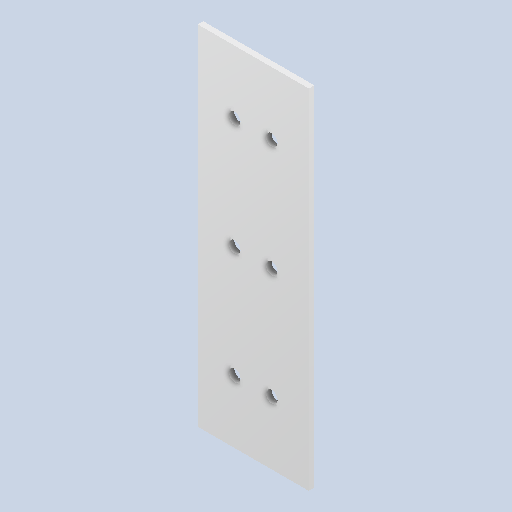
# Autodesk Inventor part: rail_rail
Saved by Autodesk Inventor 2024.1 (Build 281209000, 209)
## iProperties
Created: 2025-01-17
Part Number: rail_rail
Material: アルミニウム 6061
Document SubType Name: Sheet Metal
Designer: hibik
Density: 2.7 g/cm^3
Sheet Metal Rule: Default_mm
Appearance: アルミニウム - フラット
Author: hibik
Autodesk Inventor part; units mm, degrees
ref_plane "YZ Plane" through (0, 0, 0) normal (1, 0, 0) x (0, 1, 0)
ref_plane "XZ Plane" through (0, 0, 0) normal (0, 1, 0) x (-1, 0, 0)
ref_plane "XY Plane" through (0, 0, 0) normal (0, 0, 1) x (1, 0, 0)
sketch "スケッチ1" plane through (0, 0, 0) normal (0, 0, 1) x (1, 0, 0)
  line L0 (0, 0) -> (30, 0)
  line L1 (30, 0) -> (30, 94)
  line L2 (30, 94) -> (0, 94)
  line L3 (0, 94) -> (0, 0)
  dimension "d0" = 30
  dimension "d1" = 94
  measures "d0" distance of L2.end L1.end
  measures "d1" distance of L1.end L0.end
extrude "プレート1" add sketch "スケッチ1" along normal blind 1.5
sketch "スケッチ2" plane through (0, 0, 1.5) normal (0, 0, 1) x (1, 0, 0)
  line L0 (30, 94) -> (30, 0) projected
  circle A0 centre (10, 47) radius 1.6
  circle A1 centre (20, 47) radius 1.6
  line L1 (30, 0) -> (0, 0) projected
  line L2 (30, 94) -> (30, 0) projected
  line L3 (0, 94) -> (30, 94) projected
  line L4 (0, 0) -> (0, 94) projected
  line L5 (15, 94) -> (15, 0)
  circle A2 centre (20, 17) radius 1.6
  circle A3 centre (10, 17) radius 1.6
  circle A4 centre (20, 77) radius 1.6
  circle A5 centre (10, 77) radius 1.6
  circle A6 centre (20, 47) radius 1.6
  circle A7 centre (10, 47) radius 1.6
  point P0 (30, 47)
  dimension "d3" = 3.2
  dimension "d4" = 3.2
  dimension "d5" = 10
  dimension "d8" = 30
  dimension "d11" = 30
  constraints: 8 centre point, 3 midpoint, 2 end point, 2 vertical, 1 horizontal alignment, 1 symmetric about line, 12 other
  measures "d3" diameter of A0
  measures "d4" diameter of A1
  measures "d5" distance of A1.centre A0.centre
  measures "d8" distance of A1.centre A2.centre
  measures "d11" distance of A1.centre A4.centre
extrude "切り取り1" cut sketch "スケッチ2" against normal blind 1.5 contours A0 | A1 | A2 | A3 | A4 | A5
equation "\"d14\" = Thickness"
equation "\"d2\" = Thickness"
equation "\"BendRadius\" = Thickness"
equation "\"BendReliefWidth\" = Thickness"
equation "\"BendReliefDepth\" = 0.5 * Thickness"
equation "\"CornerReliefSize\" = 4 * Thickness"
equation "\"MinimumRemnant\" = 2 * Thickness"
equation "\"TransitionRadius\" = BendRadius"
equation "\"JacobiRadiusSize\" = BendRadius"
equation "\"GapSize\" = Thickness"
equation "\"Thickness\" = 1.5"
